Autodesk Fusion 360 part; units mm, degrees
(part 2 of 2)
sketch "Sketch12" plane through (0, 2.54, 0) normal (0, 1, 0) x (-1, 0, 0)
  line L0 (-6.35, -67.31) -> (-6.35, -73.66)
  line L1 (-6.35, -73.66) -> (158.75, -73.66)
  line L2 (158.75, -73.66) -> (158.75, -67.31)
  arc A0 (168.91, -57.15) -> (158.75, -67.31) centre (168.91, -67.31) ccw
  line L3 (168.91, -57.15) -> (175.26, -57.15)
  line L4 (175.26, -57.15) -> (175.26, 82.55)
  line L5 (175.26, 82.55) -> (168.91, 82.55)
  arc A1 (158.75, 92.71) -> (168.91, 82.55) centre (168.91, 92.71) ccw
  line L6 (158.75, 92.71) -> (158.75, 99.06)
  line L7 (158.75, 99.06) -> (-6.35, 99.06)
  line L8 (-6.35, 99.06) -> (-6.35, 92.71)
  arc A2 (-16.51, 82.55) -> (-6.35, 92.71) centre (-16.51, 92.71) ccw
  line L9 (-16.51, 82.55) -> (-22.86, 82.55)
  line L10 (-22.86, 82.55) -> (-22.86, -57.15)
  line L11 (-22.86, -57.15) -> (-16.51, -57.15)
  arc A3 (-6.35, -67.31) -> (-16.51, -57.15) centre (-16.51, -67.31) ccw
  line L12 (175.26, 82.55) -> (175.26, 74.2569) construction
  line L13 (175.26, 38.7477) -> (175.26, 30.4546) construction
  line L14 (175.26, -5.0546) -> (175.26, -13.3477) construction
  line L15 (175.26, -57.15) -> (175.26, -48.8569) construction
  line L16 (175.26, 74.2569) -> (177.8, 74.2569) construction
  line L17 (177.8, 74.2569) -> (180.8, 74.2569) construction
  line L18 (180.8, 74.2569) -> (140.8, 74.2569) construction
  line L19 (175.26, 38.7477) -> (140.8, 38.7477) construction
  line L20 (140.8, 38.7477) -> (140.8, 74.2569) construction
  line L21 (140.8, 74.2569) -> (175.26, 74.2569) construction
  line L22 (175.26, 74.2569) -> (175.26, 38.7477) construction
  line L23 (140.8, 74.2569) -> (134.45, 74.2569) construction
  line L24 (134.45, 74.2569) -> (134.45, 38.7477) construction
  line L25 (134.45, 38.7477) -> (140.8, 38.7477) construction
  line L26 (140.8, 38.7477) -> (140.8, 74.2569) construction
  line L27 (175.26, 30.4546) -> (140.8, 30.4546) construction
  line L28 (175.26, -5.0546) -> (140.8, -5.0546) construction
  line L29 (140.8, 30.4546) -> (134.45, 30.4546) construction
  line L30 (134.45, 30.4546) -> (134.45, -5.0546) construction
  line L31 (134.45, -5.0546) -> (140.8, -5.0546) construction
  line L32 (140.8, -5.0546) -> (140.8, 30.4546) construction
  line L33 (175.26, -13.3477) -> (140.8, -13.3477) construction
  line L34 (175.26, -48.8569) -> (140.8, -48.8569) construction
  line L35 (140.8, -48.8569) -> (134.45, -48.8569) construction
  line L36 (134.45, -48.8569) -> (134.45, -13.3477) construction
  line L37 (134.45, -13.3477) -> (140.8, -13.3477) construction
  line L38 (140.8, -13.3477) -> (140.8, -48.8569) construction
  line L39 (140.8, 38.7477) -> (140.8, 30.4546)
  line L40 (134.45, 38.7477) -> (134.45, 30.4546)
  line L41 (134.45, -5.0546) -> (134.45, -13.3477) construction
  line L42 (140.8, -5.0546) -> (140.8, -13.3477) construction
  line L43 (175.26, 146.05) -> (175.26, 285.75) construction
  line L44 (158.75, 302.2075) -> (123.6863, 302.2075) construction
  line L45 (175.26, 302.2075) -> (140.7922, 302.2075) construction
  line L46 (140.7922, 302.2075) -> (140.7922, 277.3917) construction
  line L47 (140.7922, 277.3917) -> (175.26, 277.3917) construction
  line L48 (175.26, 277.3917) -> (175.26, 302.2075) construction
  line L49 (158.75, 129.54) -> (139.7, 129.54) construction
  line L50 (175.26, 129.54) -> (140.7922, 129.54) construction
  line L51 (140.7922, 129.54) -> (140.7922, 154.3558) construction
  line L52 (140.7922, 154.3558) -> (175.26, 154.3558) construction
  line L53 (175.26, 154.3558) -> (175.26, 129.54) construction
  line L54 (140.7922, 277.3917) -> (140.7922, 154.3558) construction
  line L55 (140.7922, 154.3558) -> (134.4422, 154.3558) construction
  line L56 (134.4422, 154.3558) -> (134.4422, 277.3917) construction
  line L57 (134.4422, 277.3917) -> (140.7922, 277.3917) construction
  line L58 (137.6172, 154.3558) -> (137.6172, 277.3917) construction
  line L59 (134.4422, 215.8738) -> (140.7922, 215.8738) construction
  line L60 (134.4422, 154.3558) -> (134.3008, 154.2144) construction
  line L61 (134.4422, 154.3558) -> (134.2422, 154.3558) construction
  line L62 (140.7922, 277.3917) -> (140.9336, 277.5331) construction
  line L63 (140.7922, 277.3917) -> (141.3002, 277.3917) construction
  line L64 (140.9336, 277.5331) -> (134.3008, 277.5331)
  line L65 (134.3008, 277.5331) -> (134.3008, 154.2144)
  line L66 (134.3008, 154.2144) -> (140.9336, 154.2144)
  line L67 (140.9336, 154.2144) -> (140.9336, 277.5331)
  line L68 (134.3008, 277.5331) -> (131.7608, 277.5331) construction
  line L69 (131.7608, 277.5331) -> (131.7608, 280.0731) construction
  line L70 (140.9336, 154.2144) -> (143.4736, 154.2144) construction
  line L71 (143.4736, 154.2144) -> (143.4736, 151.6744) construction
  line L72 (143.4736, 151.6744) -> (131.7608, 151.6744)
  line L73 (131.7608, 151.6744) -> (131.7608, 280.0731)
  line L74 (131.7608, 280.0731) -> (143.4736, 280.0731)
  line L75 (143.4736, 280.0731) -> (143.4736, 151.6744)
  line L76 (134.45, 74.2569) -> (134.3086, 74.3983) construction
  line L77 (134.45, 74.2569) -> (134.25, 74.2569) construction
  line L78 (140.8, -48.8569) -> (140.9414, -48.9983) construction
  line L79 (140.8, -48.8569) -> (141, -48.8569) construction
  line L80 (140.9414, -48.9983) -> (134.3086, -48.9983)
  line L81 (134.3086, -48.9983) -> (134.3086, 74.3983)
  line L82 (134.3086, 74.3983) -> (140.9414, 74.3983)
  line L83 (140.9414, 74.3983) -> (140.9414, -48.9983)
  line L84 (143.4814, 76.9383) -> (140.9414, 76.9383) construction
  line L85 (140.9414, 76.9383) -> (140.9414, 74.3983) construction
  line L86 (131.7686, -51.5383) -> (134.3086, -51.5383) construction
  line L87 (134.3086, -51.5383) -> (134.3086, -48.9983) construction
  line L88 (131.7686, -51.5383) -> (143.4814, -51.5383)
  line L89 (143.4814, -51.5383) -> (143.4814, 76.9383)
  line L90 (143.4814, 76.9383) -> (131.7686, 76.9383)
  line L91 (131.7686, 76.9383) -> (131.7686, -51.5383)
  circle A4 centre (0, 92.71) radius 3.175
  circle A5 centre (0, 92.71) radius 1.25
  line L92 (-1.25, 92.71) -> (67.15, 92.71) construction
  circle A6 centre (65.9, 92.71) radius 1.25
  circle A7 centre (65.9, 92.71) radius 3.175
  circle A8 centre (69.628, 29.9607) radius 1.25
  circle A9 centre (69.628, 29.9607) radius 3.175
  line L93 (69.628, 29.9607) -> (69.628, 31.2107) construction
  circle A10 centre (69.628, 8.0607) radius 1.25
  line L94 (69.628, 8.0607) -> (69.628, 29.9607) construction
  circle A11 centre (69.628, 8.0607) radius 3.175
  line L95 (65.9, 92.71) -> (65.9, 46.71) construction
  circle A12 centre (69.628, -27.4993) radius 1.25
  circle A13 centre (69.628, -5.5993) radius 3.175
  circle A14 centre (69.628, -5.5993) radius 1.25
  circle A15 centre (69.628, -27.4993) radius 3.175
  line L96 (69.628, -27.4993) -> (69.628, -5.5993) construction
  line L97 (69.628, -5.5993) -> (69.628, -4.3493) construction
  line L98 (69.628, -63.0593) -> (69.628, -41.1593) construction
  circle A16 centre (69.628, -41.1593) radius 3.175
  circle A17 centre (69.628, -63.0593) radius 1.25
  line L99 (69.628, -41.1593) -> (69.628, -39.9093) construction
  circle A18 centre (69.628, -41.1593) radius 1.25
  circle A19 centre (69.628, -63.0593) radius 3.175
  dimension "d246" = 8.2931
  dimension "d247" = 3
  dimension "d248" = 40
  dimension "d249" = 6.35
  dimension "d253" = 123.1138
  dimension "d256" = 34.4678
  dimension "d257" = 24.8158
  dimension "d258" = 34.4678
  dimension "d259" = 24.8158
  dimension "d260" = 6.35
  dimension "d261" = 45
  dimension "d262" = 0.2
  dimension "d263" = 0.2
  dimension "d264" = 45
  dimension "d265" = 2.54
  dimension "d266" = 2.54
  dimension "d267" = 2.54
  dimension "d268" = 2.54
  dimension "d375" = 45
  dimension "d376" = 0.2
  dimension "d377" = 45
  dimension "d378" = 0.2
  dimension "d380" = 2.54
  dimension "d382" = 2.54
  dimension "d388" = 6.35
  dimension "d389" = 2.5
  dimension "d390" = 6.35
  dimension "d391" = 6.35
  dimension "d392" = 68.4
  dimension "d393" = 2.5
  dimension "d394" = 6.35
  dimension "d395" = 2.5
  dimension "d396" = 6.35
  dimension "d398" = 2.5
  dimension "d399" = 6.35
  dimension "d400" = 21.9
  dimension "d401" = 46
  dimension "d403" = 2.5
  dimension "d404" = 6.35
  dimension "d405" = 2.5
  dimension "d406" = 6.35
  dimension "d407" = 21.9
  dimension "d408" = 2.5
  dimension "d409" = 6.35
  dimension "d410" = 2.5
  dimension "d411" = 6.35
  dimension "d412" = 21.9
  constraint coincident L4.end L5.start
  constraint coincident L4 L12.end
  constraint coincident L4 L13.start
  constraint coincident L4 L13.end
  constraint coincident L4 L14.start
  constraint coincident L4 L14.end
  constraint coincident L3.end L4.start
  constraint coincident L4 L15.end
  constraint perpendicular L12 L16
  constraint perpendicular L12 L17
  constraint perpendicular L4 L18
  constraint horizontal L19
  constraint vertical L20
  constraint horizontal L21
  constraint vertical L22
  constraint horizontal L23
  constraint vertical L24
  constraint horizontal L25
  constraint vertical L26
  constraint perpendicular L13 L27
  constraint perpendicular L14 L28
  constraint horizontal L29
  constraint vertical L30
  constraint horizontal L31
  constraint vertical L32
  constraint perpendicular L32 L33
  constraint perpendicular L15 L34
  constraint horizontal L35
  constraint vertical L36
  constraint horizontal L37
  constraint vertical L38
  constraint perpendicular L29 L39
  constraint perpendicular L29 L40
  constraint perpendicular L37 L41
  constraint perpendicular L33 L42
  constraint vertical L43
  constraint horizontal L44
  constraint horizontal L45
  constraint vertical L46
  constraint horizontal L47
  constraint vertical L48
  constraint horizontal L49
  constraint horizontal L50
  constraint vertical L51
  constraint horizontal L52
  constraint vertical L53
  constraint perpendicular L54 L55
  constraint parallel L54 L56
  constraint parallel L55 L57
  constraint perpendicular L52 L54
  constraint midpoint L55 L58.start
  constraint midpoint L57 L58.end
  constraint midpoint L56 L59.start
  constraint midpoint L54 L59.end
  constraint horizontal L61
  constraint horizontal L63
  constraint horizontal L64
  constraint vertical L65
  constraint horizontal L66
  constraint vertical L67
  constraint perpendicular L65 L68
  constraint perpendicular L68 L69
  constraint perpendicular L67 L70
  constraint perpendicular L70 L71
  constraint horizontal L72
  constraint vertical L73
  constraint horizontal L74
  constraint vertical L75
  constraint horizontal L77
  constraint horizontal L79
  constraint horizontal L80
  constraint vertical L81
  constraint horizontal L82
  constraint vertical L83
  constraint horizontal L84
  constraint vertical L85
  constraint horizontal L86
  constraint vertical L87
  constraint horizontal L88
  constraint vertical L89
  constraint horizontal L90
  constraint vertical L91
  constraint concentric A4 A5
  constraint coincident A5 L92.start
  constraint horizontal L92
  constraint coincident L92.end A6
  constraint concentric A6 A7
  constraint concentric A8 A9
  constraint coincident A8.centre A9.centre
  constraint coincident A8 L93.end
  constraint vertical L93
  constraint coincident A10.centre L94.start
  constraint coincident A6.centre A7.centre
  constraint perpendicular L92 L95
  constraint concentric A13 A14
  constraint coincident A13.centre A14.centre
  constraint coincident L97.end A14
  constraint vertical L97
  constraint coincident A12.centre A15.centre
  constraint concentric A16 A18
  constraint coincident L98.end A16.centre
  constraint coincident L99.end A18
  constraint vertical L99
  constraint coincident L98.start A17.centre
  measures "d246" distance of L4.end L12.end
  measures "d247" distance of L16.end L17.end
  measures "d248" distance of L17.end L18.end
  measures "d249" distance of L18.end L23.end
  measures "d253" distance of L23.end L35.end
  measures "d256" distance of L45.start L45.end
  measures "d257" distance of L45.start L47.end
  measures "d258" distance of L50.start L50.end
  measures "d259" distance of L50.start L52.end
  measures "d260" distance of L46.end L56.end
  measures "d261" angle of L60 L61
  measures "d262" distance of L55.end L60.end
  measures "d263" distance of L46.end L62.end
  measures "d264" angle of L62 L63
  measures "d265" distance of L64.end L68.end
  measures "d266" distance of L68.end L69.end
  measures "d267" distance of L66.end L70.end
  measures "d268" distance of L70.end L71.end
  measures "d375" angle of L76 L77
  measures "d376" distance of L23.end L76.end
  measures "d377" angle of L78 L79
  measures "d378" distance of L34.end L78.end
  measures "d380" distance of L82.end L84.end
  measures "d382" distance of L80.end L86.end
  measures "d388" diameter of A4
  measures "d389" diameter of A5
  measures "d390" distance of L7 A4.centre
  measures "d391" distance of L8 A4.centre
  measures "d392" distance of L92.start L92.end
  measures "d393" diameter of A6
  measures "d394" diameter of A7
  measures "d395" diameter of A8
  measures "d396" diameter of A9
  measures "d398" diameter of A10
  measures "d399" diameter of A11
  measures "d400" distance of A8.centre A10.centre
  measures "d401" distance of A6.centre L95.end
  measures "d403" diameter of A14
  measures "d404" diameter of A13
  measures "d405" diameter of A12
  measures "d406" diameter of A15
  measures "d407" distance of A13.centre A12.centre
  measures "d408" diameter of A18
  measures "d409" diameter of A16
  measures "d410" diameter of A17
  measures "d411" diameter of A19
  measures "d412" distance of L98.end L98.start
extrude "Extrude22" add sketch "Sketch12" along normal blind 8.89 contours L72 L73 L74 L75 bodies 2
extrude "Extrude23" cut sketch "Sketch10" against normal blind 5.08 contours A5 L57 L99 | A5 L99 | A3 L78 L97 | A3 A30 L78 L82 L97 | A3 L82 | A5 A18 L56 L57 | A30 | A3 L74 A30 L78 L97 | A3 A30 L82 L83 | A5 A18 L57 L59 | A2 L37 L99 | A2 L99 | A5 L56 | A18 | A3 L74 A30 L83 | A3 L74 | A3 L83 | A0 L85 | A0 L85 A36 L89 L97 | A0 L89 L97 | A5 L59 | A2 L33 A9 L37 | A5 A18 L55 L56 | A5 A18 L55 L59 | A2 A9 L35 L37 | A0 L85 A36 L94 | A36 | A0 A36 L89 L93 L97 | A2 L33 | A9 | A5 L55 | A2 L35 | A0 L94 | A0 A36 L93 L94 | A0 L93 | A2 L29 L33 A9 | A2 L29 A9 L35 | A2 L29 | A1 L40 | A1 L40 A15 L46 | A1 L40 L44 A15 | A1 L46 | A15 | A1 L44 | A1 A15 L46 L48 | A1 L44 A15 L48 | A1 L48 | A4 L67 | A4 L63 A24 L67 | A4 A24 L67 L71 | A4 L63 | A24 | A4 L71 | A4 L63 A24 L72 | A4 A24 L71 L72 | A4 L72 | A6 | A7 | A8 | A10 | A11 | A12 | A13 | A14 | A16 | A17 | A19 | A20 | A21 | A22 | A23 | A25 | A26 | A27 | A28 | A29 | A31 | A32 | A33 | A34 | A35 | A37 | A38 | A39 | A40 | A41 bodies 1
extrude "Extrude24" add sketch "Sketch12" along normal blind 7.62 contours L88 L89 L90 L91 bodies 1
sketch "Sketch13" plane through (22.86, 0, 0) normal (-1, 0, 0) x (0, 0, 1)
  line L0 (-63.5, 99.06) -> (-57.15, 99.06)
  line L1 (-57.15, 99.06) -> (-57.15, 2.54)
  line L2 (-57.15, 2.54) -> (82.55, 2.54)
  line L3 (82.55, 2.54) -> (82.55, 99.06)
  line L4 (82.55, 99.06) -> (88.9, 99.06)
  line L5 (88.9, 99.06) -> (88.9, 101.6)
  line L6 (88.9, 101.6) -> (-63.5, 101.6)
  line L7 (-63.5, 101.6) -> (-63.5, 99.06)
  line L8 (-57.15, 99.06) -> (82.55, 99.06) construction
  line L9 (-57.15, 2.54) -> (-57.15, 99.06) construction
  line L10 (-57.15, 50.8) -> (33.02, 50.8) construction
  line L11 (12.7, 99.06) -> (12.7, 2.54) construction
  circle A0 centre (12.7, 50.8) radius 10.5
  dimension "d385" = 21
  constraint coincident L0.end L1.start
  constraint coincident L3.end L4.start
  constraint coincident L1.end L2.start
  constraint midpoint L9 L10.start
  constraint perpendicular L9 L10
  constraint midpoint L8 L11.start
  constraint midpoint L2 L11.end
  constraint midpoint L11 A0.centre
  measures "d385" diameter of A0
extrude "Extrude25" cut sketch "Sketch13" against normal blind 10.16 contours A0 bodies 1
extrude "Extrude26" add sketch "Sketch12" along normal blind 5.08 contours A4 | A7 | A9 | A11 | A13 | A15 | A16 | A19 bodies 1
equation "d201 = 0.3265 in + 0.699 in"
equation "d202 = 0.368 in + 0.699 in"
equation "d204 = 0.3265 in + 0.699 in"
equation "d205 = 0.368 in + 0.699 in"
equation "d206 = 0.368 in + 0.699 in"
equation "d224 = 6.4 mm + 1.5 mm"
